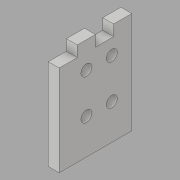
# Autodesk Inventor part: e_arm holder 2
Saved by Autodesk Inventor 2019 (Build 230136000, 136)
## iProperties
Created: 2021-11-01
Part Number: e_arm holder 2
Material: Generic
Document SubType Name: Modeling
Designer: Mohamed
Density: 1 g/cm^3
Appearance: Default
Author: Mohamed
Autodesk Inventor part; units mm, degrees
ref_plane "YZ Plane" through (0, 0, 0) normal (1, 0, 0) x (0, 1, 0)
ref_plane "XZ Plane" through (0, 0, 0) normal (0, 1, 0) x (-1, 0, 0)
ref_plane "XY Plane" through (0, 0, 0) normal (0, 0, 1) x (1, 0, 0)
sketch "Sketch1" plane through (0, 0, 0) normal (1, 0, 0) x (0, 1, 0)
  line L0 (0, 0) -> (56, 0)
  line L1 (56, 0) -> (56, -40)
  line L2 (56, -40) -> (0, -40)
  line L3 (0, -40) -> (0, 0)
  dimension "d0" = 56
  dimension "d1" = 40
  constraints: 8 end point, 2 parallel, 1 horizontal, 1 perpendicular
  measures "d0" distance of L1.end L2.end
  measures "d1" distance of L0.end L1.end
extrude "Extrusion1" add sketch "Sketch1" along normal blind 6
sketch "Sketch2" plane through (6, 0, 0) normal (1, 0, 0) x (0, 0, -1)
  line L0 (40, 56) -> (0, 56) projected
  line L1 (40, 56) -> (30, 56)
  line L2 (30, 56) -> (20, 56)
  line L3 (20, 56) -> (20, 50)
  line L4 (20, 50) -> (30, 50)
  line L5 (30, 50) -> (30, 56)
  point P0 (0, 0)
  dimension "d4" = 10
  dimension "d5" = 10
  dimension "d6" = 6
  constraints: 10 end point, 2 parallel, 1 horizontal, 1 perpendicular, 1 point on line
  measures "d4" distance of L0.start L1.end
  measures "d5" distance of L4.end L3.end
  measures "d6" distance of L3.end L2.end
extrude "Extrusion2" cut sketch "Sketch2" against normal blind 6
pattern_linear "Rectangular Pattern1" count 2 spacing 20 along (0, 0, 1) of "Extrusion2"
sketch "Sketch3" plane through (6, 0, 0) normal (1, 0, 0) x (0, 0, -1)
  line L0 (30, 50) -> (30, 56) projected
  circle A0 centre (15, 41.5) radius 3
  circle A1 centre (29, 41.5) radius 3
  circle A2 centre (15, 19.5) radius 3
  circle A3 centre (29, 19.5) radius 3
  point P0 (0, 0)
  dimension "d14" = 6
  dimension "d16" = 6
  dimension "d18" = 6
  dimension "d19" = 6
  constraints: 4 centre point
  measures "d14" diameter of A0
  measures "d16" diameter of A1
  measures "d18" diameter of A2
  measures "d19" diameter of A3
extrude "Extrusion3" cut sketch "Sketch3" against normal blind 6
body "Solid1"
